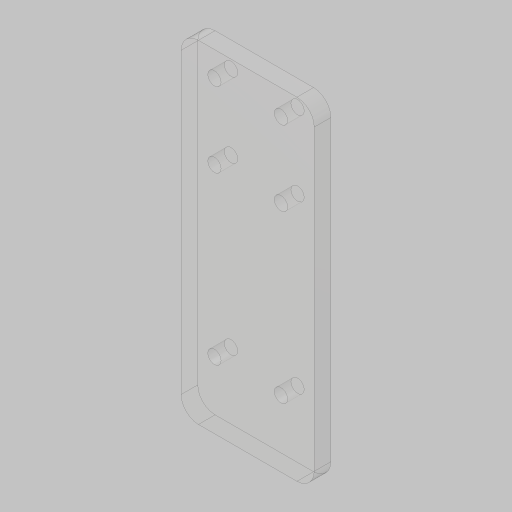
# Autodesk Inventor part: CL7-GB-003
Saved by Autodesk Inventor 2023.5 (Build 275446000, 446)
## iProperties
Created: 2025-03-18
Part Number: CL7-GB-003
Material: Polycarbonate, Clear
Document SubType Name: Modeling
Designer: slick
Density: 1.2 g/cm^3
Appearance: Polycarbonate - Clear
Author: slick
Autodesk Inventor part; units mm, degrees
ref_plane "YZ Plane" through (0, 0, 0) normal (1, 0, 0) x (0, 1, 0)
ref_plane "XZ Plane" through (0, 0, 0) normal (0, 1, 0) x (-1, 0, 0)
ref_plane "XY Plane" through (0, 0, 0) normal (0, 0, 1) x (1, 0, 0)
sketch "Sketch1" plane through (0, 0, 0) normal (0, 0, 1) x (1, 0, 0)
  line L0 (25.4, -63.5) -> (-25.4, -63.5)
  line L1 (-25.4, -63.5) -> (-25.4, 63.5)
  line L2 (-25.4, 63.5) -> (25.4, 63.5)
  line L3 (25.4, 63.5) -> (25.4, -63.5)
  line L4 (25.4, -63.5) -> (-25.4, 63.5) construction
  line L5 (-25.4, -63.5) -> (25.4, 63.5) construction
  line L6 (-12.7, 53.975) -> (12.7, 53.975) construction
  point P0 (0, 0)
  point P1 (-12.7, 25.4)
  point P2 (12.7, 25.4)
  point P3 (12.7, -38.1)
  point P4 (-12.7, -38.1)
  point P5 (0, 53.975)
  point P6 (0, 63.5)
  dimension "d0" = 50.8
  dimension "d1" = 127
  dimension "d2" = 9.525
  dimension "d3" = 25.4
  dimension "d4" = 38.1
  dimension "d5" = 63.5
  constraints: 14 end point, 5 vertical alignment, 4 midpoint, 3 horizontal alignment, 2 horizontal, 2 parallel, 1 perpendicular
  measures "d0" distance of L1.end L2.end
  measures "d1" distance of L0.end L1.end
  measures "d2" distance from line of L2 L6.start
  measures "d3" distance of L6.end L6.start
  measures "d4" distance from line of point (-12.7, 25.4) L2
  measures "d5" distance of point (-12.7, -38.1) point (-12.7, 25.4)
extrude "Extrusion1" add sketch "Sketch1" along normal blind 6.35
hole "Hole1" at (-12.7, 53.975, 0) at (12.7, 53.975, 0) at (-12.7, 25.4, 0) at (12.7, 25.4, 0) at (12.7, -38.1, 0) at (-12.7, -38.1, 0) direction (0, 0, 1) diameter 5.1054 end through all clearance for "Flat Head Machine Screw (82)" size "#10" standard "Ansi Unified Screw Threads"
fillet "Fillet1" radius 6.604 4 edges at (25.4, 63.5, 3.175) (-25.4, 63.5, 3.175) (25.4, -63.5, 3.175) (-25.4, -63.5, 3.175)
body "Solid1"
